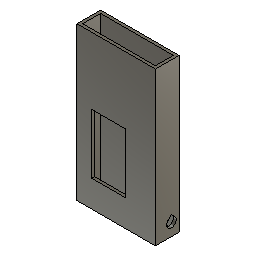
openepaper_diy_ap_doosje v1 (Autodesk Fusion 360 design; units mm, degrees)
Autodesk Fusion 360 part; units mm, degrees
note: some values were not read from the file. Set by a fixed rule: which face or edge a step refers to.
sketch "Sketch1" plane through (0, 0, 0) normal (0, 0, 1) x (1, 0, 0)
  line L0 (0, 0) -> (30.5, 0)
  line L1 (30.5, 0) -> (30.5, 7.5)
  line L2 (30.5, 7.5) -> (0, 7.5)
  line L3 (0, 7.5) -> (0, 0)
  dimension "d1" = 30.5
  dimension "d2" = 7.5
  constraint horizontal L0
  constraint vertical L1
  constraint horizontal L2
  constraint vertical L3
  constraint coincident L0.start L3.end
  measures "d1" distance of L0.start L0.end
  measures "d2" distance of L0.start L2.end
extrude "Extrude1" add sketch "Sketch1" along normal blind 63
shell "Shell1" thickness 1.2 outward yes removed faces 1 at (10.1667, 5, 63)
sketch "Sketch2" plane through (0, -1.2, 0) normal (0, -1, 0) x (1, 0, 0)
  line L0 (-1.2, -1.2) -> (31.7, -1.2)
  line L1 (31.7, -1.2) -> (31.7, 63)
  line L2 (31.7, 63) -> (-1.2, 63)
  line L3 (-1.2, 63) -> (-1.2, -1.2)
  line L4 (5, 10) -> (19, 10)
  line L5 (19, 10) -> (19, 35)
  line L6 (19, 35) -> (5, 35)
  line L7 (5, 35) -> (5, 10)
  dimension "d6" = 14
  dimension "d7" = 25
  dimension "d8" = 5
  dimension "d9" = 10
  constraint horizontal L4
  constraint vertical L5
  constraint horizontal L6
  constraint vertical L7
  measures "d6" distance of L4.start L4.end
  measures "d7" distance of L4.end L5.end
  measures "d8" distance of origin L7
  measures "d9" distance of origin L4
extrude "Extrude2" cut sketch "Sketch2" against normal up to surface (1.2 mm away) contours L4 L5 L6 L7
sketch "Sketch3" plane through (0, 0, -1.2) normal (0, 0, -1) x (1, 0, 0)
  line L0 (-1.2, 1.2) -> (-1.2, -8.7)
  line L1 (-1.2, -8.7) -> (31.7, -8.7)
  line L2 (31.7, -8.7) -> (31.7, 1.2)
  line L3 (31.7, 1.2) -> (-1.2, 1.2)
  line L4 (0, -7.5) -> (0, 0)
  circle A0 centre (15.25, -5.75) radius 1.75
  circle A1 centre (9.25, -5.75) radius 1.75
  line L5 (15.25, -4) -> (9.25, -4)
  line L6 (9.25, -7.5) -> (15.25, -7.5)
  line L7 (0, -7.5) -> (14.7068, -7.5) construction
  dimension "d12" = 1.2
  dimension "d13" = 3.5
  dimension "d14" = 6
  dimension "d16" = 9.25
  constraint equal A0 A1
  constraint coincident A0 L5.start
  constraint coincident A1 L5.end
  constraint tangent A0 L5
  constraint tangent A1 L5
  constraint horizontal L5
  constraint coincident A1 L6.start
  constraint coincident A0 L6.end
  constraint tangent A0 L6
  constraint tangent A1 L6
  constraint perpendicular L4 L7
  constraint coincident L4.start L7.start
  constraint collinear L6 L7
  measures "d12" distance of L0 L4
  measures "d13" distance of L5 L6
  measures "d14" distance of A0.centre A1.centre
  measures "d16" distance of L4 A1.centre
extrude "Extrude3" cut sketch "Sketch3" against normal up to surface (1.2 mm away) contours A0 | A0 A1 L5 L6 | A1
sketch "Sketch5" plane through (31.7, 0, 0) normal (1, 0, 0) x (0, 1, 0)
  line L0 (-1.2, -1.2) -> (8.7, -1.2)
  line L1 (8.7, -1.2) -> (8.7, 63)
  line L2 (8.7, 63) -> (-1.2, 63)
  line L3 (-1.2, 63) -> (-1.2, -1.2)
  circle A0 centre (5.5, 4) radius 2
  line L4 (5.5, 4) -> (5.5, 11.0794) construction
  line L5 (5.5, 6.8284) -> (4.0858, 5.4142)
  line L6 (5.5, 6.8284) -> (6.9142, 5.4142)
  dimension "d19" = 4
  dimension "d20" = 1.2
  dimension "d21" = 3.2
  dimension "d22" = 5.2
  constraint coincident A0.centre L4.start
  constraint parallel L1 L4
  constraint coincident L4 L5.start
  constraint coincident A0 L5.end
  constraint coincident A0 L6.end
  constraint perpendicular L5 L6
  constraint tangent A0 L5
  constraint tangent A0 L6
  measures "d19" diameter of A0
  measures "d20" distance of origin L3
  measures "d21" distance of L1 A0.centre
  measures "d22" distance of L0 A0.centre
extrude "Extrude4" cut sketch "Sketch5" against normal up to surface (1.2 mm away) contours A0 | A0 L5 L6
equation "d16 = 7.5 mm + ( d13 / 2 )"
equation "d21 = ( d19 / 2 ) + d20"
equation "d22 = d20 + ( d19 / 2 ) + 2 mm"
